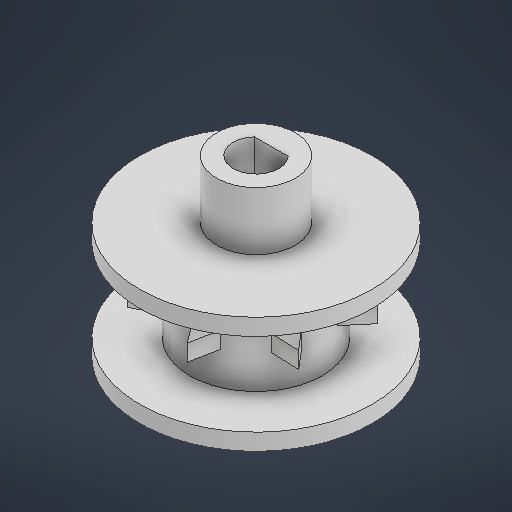
# Autodesk Inventor part: Part1
Saved by Autodesk Inventor 2026.2 (Build 302298000, 298)
## iProperties
Created: 2026-04-06
Part Number: Part1
Material: Generic
Document SubType Name: Modeling
Designer: Brian Wang
Density: 1 g/cm^3
Appearance: Default
Author: Brian Wang
Autodesk Inventor part; units mm, degrees
ref_plane "YZ Plane" through (0, 0, 0) normal (1, 0, 0) x (0, 1, 0)
ref_plane "XZ Plane" through (0, 0, 0) normal (0, 1, 0) x (-1, 0, 0)
ref_plane "XY Plane" through (0, 0, 0) normal (0, 0, 1) x (1, 0, 0)
sketch "Sketch1" plane through (0, 0, 0) normal (0, 1, 0) x (-1, 0, 0)
  line L0 (0, 0) -> (13.4559, 0) construction
  line L1 (7.8785, 1.3892) -> (11, 0)
  line L2 (7.8785, -1.3892) -> (11, 0)
  line L3 (5.9982, 5.2935) -> (6.8584, 8.6001)
  line L4 (3.826, 7.0258) -> (6.8584, 8.6001)
  line L5 (-0.3988, 7.9901) -> (-2.4477, 10.7242)
  line L6 (-3.1075, 7.3718) -> (-2.4477, 10.7242)
  line L7 (-6.4955, 4.6699) -> (-9.9107, 4.7727)
  line L8 (-7.701, 2.1667) -> (-9.9107, 4.7727)
  line L9 (-7.701, -2.1667) -> (-9.9107, -4.7727)
  line L10 (-6.4955, -4.6699) -> (-9.9107, -4.7727)
  line L11 (-3.1075, -7.3718) -> (-2.4477, -10.7242)
  line L12 (-0.3988, -7.9901) -> (-2.4477, -10.7242)
  line L13 (3.826, -7.0258) -> (6.8584, -8.6001)
  line L14 (5.9982, -5.2935) -> (6.8584, -8.6001)
  arc A0 (7.8785, 1.3892) -> (5.9982, 5.2935) centre (0, 0) ccw
  arc A1 (5.9982, -5.2935) -> (7.8785, -1.3892) centre (0, 0) ccw
  arc A2 (-0.3988, -7.9901) -> (3.826, -7.0258) centre (0, 0) ccw
  arc A3 (-6.4955, -4.6699) -> (-3.1075, -7.3718) centre (0, 0) ccw
  arc A4 (-7.701, 2.1667) -> (-7.701, -2.1667) centre (0, 0) ccw
  arc A5 (3.826, 7.0258) -> (-0.3988, 7.9901) centre (0, 0) ccw
  arc A6 (-3.1075, 7.3718) -> (-6.4955, 4.6699) centre (0, 0) ccw
  dimension "d10" = 360
  constraints: 30 end point, 14 point on circle, 7 centre point, 1 coincident, 1 horizontal, 1 point on line, 36 other
extrude "Extrusion1" add sketch "Sketch1" along normal blind 2
sketch "Sketch2" plane through (0, 2, 0) normal (0, 1, 0) x (1, 0, 0)
  circle A0 centre (0, 0) radius 8
  constraints: 1 centre point, 1 coincident
extrude "Extrusion2" add sketch "Sketch2" along normal blind 4
sketch "Sketch3" plane through (0, 0, 0) normal (0, -1, 0) x (1, 0, 0)
  circle A0 centre (0, 0) radius 8
  constraints: 1 centre point, 1 coincident
extrude "Extrusion3" add sketch "Sketch3" along normal blind 4
sketch "Sketch4" plane through (0, 6, 0) normal (0, 1, 0) x (1, 0, 0)
  circle A0 centre (0, 0) radius 14
  dimension "d18" = 28
  constraints: 1 centre point, 1 coincident
  measures "d18" diameter of A0
sketch "Sketch5" plane through (0, -4, 0) normal (0, -1, 0) x (1, 0, 0)
  circle A0 centre (0, 0) radius 14
  dimension "d19" = 28
  constraints: 1 centre point, 1 coincident
  measures "d19" diameter of A0
extrude "Extrusion4" add sketch "Sketch5" along normal blind 2
extrude "Extrusion5" add sketch "Sketch4" along normal blind 2
sketch "Sketch6" plane through (0, 8, 0) normal (0, 1, 0) x (1, 0, 0)
  arc A0 (-2.0347, 1.85) -> (2.0347, 1.85) centre (0, 0) ccw
  line L0 (-2.0347, 1.85) -> (2.0347, 1.85)
  dimension "d24" = 5.5
  constraints: 2 end point, 2 point on circle, 1 centre point, 1 coincident, 1 horizontal
  measures "d24" diameter of A0
extrude "Extrusion6" cut sketch "Sketch6" against normal through all
sketch "Sketch7" plane through (0, 8, 0) normal (0, 1, 0) x (1, 0, 0)
  arc A0 (-2.0347, 1.85) -> (2.0347, 1.85) centre (0, 0) ccw projected
  circle A1 centre (0, 0) radius 4.75
  line L0 (-2.0347, 1.85) -> (2.0347, 1.85) projected
  arc A2 (-2.0347, 1.85) -> (2.0347, 1.85) centre (0, 0) ccw
  line L1 (2.0347, 1.85) -> (-2.0347, 1.85)
  dimension "d28" = 9.5
  constraints: 2 centre point, 2 end point, 2 point on circle, 1 coincident, 1 collinear, 1 concentric
  measures "d28" diameter of A1
extrude "Extrusion7" add sketch "Sketch7" along normal blind 7
body "Solid1"
